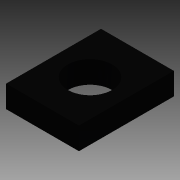
# Autodesk Inventor part: Fixture_Airpot_Support_3
Saved by Autodesk Inventor 2015 (Build 190159000, 159)
## iProperties
Created: 2014-12-16
Part Number: Fixture_Airpot_Support_3
Material: Generic
Document SubType Name: Modeling
Designer: amarschn
Density: 1 g/cm^3
Appearance: Anodized - Black
Author: amarschn
Autodesk Inventor part; units mm, degrees
ref_plane "YZ Plane" through (0, 0, 0) normal (1, 0, 0) x (0, 1, 0)
ref_plane "XZ Plane" through (0, 0, 0) normal (0, 1, 0) x (-1, 0, 0)
ref_plane "XY Plane" through (0, 0, 0) normal (0, 0, 1) x (1, 0, 0)
sketch "Sketch1" plane through (0, 0, 0) normal (0, 1, 0) x (-1, 0, 0)
  line L0 (-20.955, -27.305) -> (20.955, -27.305)
  line L1 (20.955, -27.305) -> (20.955, 27.305)
  line L2 (20.955, 27.305) -> (-20.955, 27.305)
  line L3 (-20.955, 27.305) -> (-20.955, -27.305)
  line L4 (-20.955, -27.305) -> (20.955, 27.305) construction
  line L5 (20.955, -27.305) -> (-20.955, 27.305) construction
  circle A0 centre (0, 0) radius 12.7
  dimension "d0" = 54.61
  dimension "d1" = 41.91
  dimension "d2" = 25.4
  constraints: 12 end point, 2 midpoint, 2 parallel, 1 centre point, 1 coincident, 1 horizontal, 1 perpendicular
  measures "d0" distance of L0.end L1.end
  measures "d1" distance of L1.end L2.end
  measures "d2" diameter of A0
extrude "Extrusion1" add sketch "Sketch1" along normal blind 12.7
body "Solid1"
